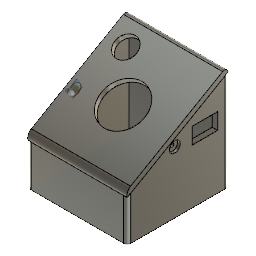
AntiThief_yanweibo (Autodesk Fusion 360 design; units mm, degrees)
Autodesk Fusion 360 part; units mm, degrees
sketch "Sketch1" plane through (0, 0, 0) normal (0, 1, 0) x (1, 0, 0) in component "Case"
  line L0 (27.5, 11.5) -> (-27.5, 11.5)
  line L1 (-27.5, 11.5) -> (-27.5, -11.5)
  line L2 (-27.5, -11.5) -> (27.5, -11.5)
  line L3 (27.5, -11.5) -> (27.5, 11.5)
  line L4 (27.5, 11.5) -> (-27.5, -11.5) construction
  line L5 (-27.5, 11.5) -> (27.5, -11.5) construction
  dimension "d1" = 55
  dimension "d2" = 23
  constraint perpendicular L0 L1
  constraint parallel L0 L2
  constraint parallel L1 L3
  constraint horizontal L0
  constraint coincident L4 origin
  constraint coincident L5 origin
  measures "d1" distance of L1.end L2.end
  measures "d2" distance of L0.end L1.end
extrude "Extrude1" add sketch "Sketch1" along normal blind 56 contours L0 L1 L2 L3 picked at (-9.166667, -3.833333) makes body 1 in component "Case"
sketch "Sketch3" plane through (0, 0, 11.5) normal (0, 0, 1) x (-1, 0, 0) in component "Case"
  line L0 (27.5, 0) -> (-27.5, 0)
  line L1 (-27.5, 0) -> (-27.5, -56)
  line L2 (-27.5, -56) -> (27.5, -56)
  line L3 (27.5, -56) -> (27.5, 0)
  line L4 (24.5, -53) -> (24.5, -3)
  line L5 (24.5, -3) -> (-24.5, -3)
  line L6 (-24.5, -3) -> (-24.5, -53)
  line L7 (-24.5, -53) -> (24.5, -53)
  dimension "d7" = -3
extrude "Extrude2" cut sketch "Sketch3" against normal blind 20 contours L4 L5 L6 L7 picked at (-8.166667, -36.333333) bodies 1 in component "Case"
draft "Draft1" angle 30 neutral plane through (0, 0, 0) pull (0, -1, 0) 1 faces at (-26.5, 36.333333, 11.5) on bodies 1 in component "Case"
sketch "Sketch1 (2)" plane through (0, -4.979646, 8.625) normal (0, -0.5, 0.866025) x (1, 0, 0) in component "Top"
  line L0 (-24.5, 9.214102) -> (-24.5, 66.949129)
  line L1 (-24.5, 66.949129) -> (24.5, 66.949129)
  line L2 (24.5, 66.949129) -> (24.5, 9.214102)
  line L3 (24.5, 9.214102) -> (-24.5, 9.214102)
  line L4 (-27.5, 5.75) -> (27.5, 5.75)
  line L5 (27.5, 5.75) -> (27.5, 70.41323)
  line L6 (27.5, 70.41323) -> (-27.5, 70.41323)
  line L7 (-27.5, 70.41323) -> (-27.5, 5.75)
extrude "Extrude1'" add sketch "Sketch1 (2)" along normal blind 3 separate body contours L4 L5 L6 L7 picked at (-8.166667, 6.904701) makes body 2 in component "Top"
fillet "Fillet1" radius 2 4 edges at (27.5, 56, 16.165808) (27.5, 0, 0) (-27.5, 0, 0) (-27.5, 56, 16.165808) on bodies 1 in component "Case"
fillet "Fillet1'" radius 4 1 edges at (0, -1.5, 14.098076) on bodies 2 in component "Top"
fillet "Fillet2" radius 2 1 edges at (0, 54.5, 46.429691) on bodies 2 in component "Top"
sketch "Sketch5" plane through (0, 0, -8.5) normal (0, 0, 1) x (-1, 0, 0) in component "Case"
  line L0 (-24.5, -53) -> (24.5, -53)
  line L1 (24.5, -53) -> (24.5, -3)
  line L2 (24.5, -3) -> (-24.5, -3)
  line L3 (-24.5, -3) -> (-24.5, -53)
  line L4 (-25, -30) -> (25, -30)
  line L5 (25, -30) -> (25, -33)
  line L6 (25, -33) -> (-25, -33)
  line L7 (-25, -33) -> (-25, -30)
  line L8 (-25, -30) -> (25, -33) construction
  line L9 (25, -30) -> (-25, -33) construction
  line L10 (-25.5, 0) -> (25.5, 0)
  line L11 (-25.5, -56) -> (25.5, -56)
  point P0 (0, -31.5)
  dimension "d15" = 3
  dimension "d16" = 50
  dimension "d17" = 30
  dimension "d18" = 23
  constraint perpendicular L4 L5
  constraint parallel L4 L6
  constraint parallel L5 L7
  constraint horizontal L4
  constraint coincident L8 P0
  constraint coincident L9 P0
  measures "d15" distance of L4.end L5.end
  measures "d16" distance of L5.end L6.end
  measures "d17" distance of L4 L10
  measures "d18" distance of L6.end L11
extrude "Extrude3" add sketch "Sketch5" along normal blind 10 contours L1 L3 L4 L6 picked at (-8.166667, -31) bodies 1 in component "Case"
sketch "Sketch6" plane through (27.5, 0, 0) normal (1, 0, 0) x (0, 1, 0) in component "Case"
  line L0 (2, 12.654701) -> (2, -11.5)
  line L1 (2, -11.5) -> (54, -11.5)
  line L2 (54, -11.5) -> (54, 42.676915)
  line L3 (54, 42.676915) -> (2, 12.654701)
  circle A0 centre (26.320508, 22.654701) radius 3
  line L4 (36, 27.665808) -> (50, 27.665808)
  line L5 (50, 27.665808) -> (50, 18.665808)
  line L6 (50, 18.665808) -> (36, 18.665808)
  line L7 (36, 18.665808) -> (36, 27.665808)
  dimension "d21" = 6
  dimension "d22" = 3.5
  dimension "d23" = 10
  dimension "d92" = 14
  dimension "d93" = 9
  dimension "d94" = 18
  dimension "d95" = 4
  constraint horizontal L4
  constraint vertical L5
  constraint horizontal L6
  constraint vertical L7
  measures "d21" diameter of A0
extrude "Extrude6" cut sketch "Sketch6" against normal blind 3 contours L4 L5 L6 L7 picked at (40.666667, 21.665808) bodies 1 in component "Case"
hole "Hole2" at (27.5, 26.320508, 22.654701) direction (-1, 0, 0) diameter 2 depth 6 tip angle 118 bodies 1 in component "Case"
extrude "Extrude4" cut sketch "Sketch6" against normal blind 1.5 contours A0 picked at (26.245778, 23.519244) bodies 1 in component "Case"
sketch "Sketch8" plane through (-27.5, 0, 0) normal (-1, 0, 0) x (0, -1, 0) in component "Case"
  line L0 (-54, 42.676915) -> (-54, -11.5)
  line L1 (-54, -11.5) -> (-2, -11.5)
  line L2 (-2, -11.5) -> (-2, 12.654701)
  line L3 (-2, 12.654701) -> (-54, 42.676915)
  circle A0 centre (-26.320508, 22.654701) radius 3
  line L4 (-21.944825, 24.169851) -> (-24.944825, 18.973698)
  line L5 (-24.944825, 18.973698) -> (-30.140978, 21.973698)
  line L6 (-30.140978, 21.973698) -> (-27.140978, 27.169851)
  line L7 (-30.140978, 21.973698) -> (-24.125026, 21.973698) construction
  line L8 (-27.140978, 27.169851) -> (-21.944825, 24.169851)
  dimension "d29" = 6
  dimension "d30" = 10
  dimension "d31" = 3.5
  dimension "d53" = 6
  dimension "d54" = 6
  dimension "d55" = 60
  dimension "d56" = 6
  constraint perpendicular L3 L4
  constraint perpendicular L4 L5
  constraint horizontal L7
  measures "d29" diameter of A0
  measures "d55" angle of L6 L7
hole "Hole1" at (-27.5, 26.320508, 22.654701) direction (1, 0, 0) diameter 2 depth 6 tip angle 118 bodies 1 in component "Case"
extrude "Extrude5" cut sketch "Sketch8" against normal blind 1.5 contours A0 L6 | A0 L5 L6 | A0 L5 picked at (-28.923464, 24.10138) picked at (-27.239065, 23.000716) picked at (-27.238076, 20.214879) bodies 1 in component "Case"
sketch "Sketch2" plane through (-24.5, 0, 0) normal (1, 0, 0) x (0, 1, 0) in component "Top"
  arc A0 (1.854102, 16.034568) -> (1.510476, 15.811981) centre (3.854102, 12.570466) ccw
  line L0 (1.510476, 15.811981) -> (3, 13.232051)
  line L1 (3, 13.232051) -> (53, 42.099564)
  line L2 (53, 42.099564) -> (51.5, 44.69764)
  line L3 (51.5, 44.69764) -> (1.854102, 16.034568)
extrude "Extrude2'" add sketch "Sketch2" along normal blind 44 contours A0 L0 L1 L2 L3 picked at (19.284701, 23.788728) bodies 2 in component "Top"
extrude "拉伸8" add 1 faces at (19.5, 19.284701, 23.788728) along direction (1, 0, 0) blind 5 on bodies 2 bodies 2 in component "Top"
sketch "Sketch7" plane through (0, -4.979646, 8.625) normal (0, 0.5, -0.866025) x (-1, 0, 0) in component "Top"
  line L0 (27.5, 5.75) -> (27.5, 70.41323)
  line L1 (27.5, 70.41323) -> (-27.5, 70.41323)
  line L2 (-27.5, 70.41323) -> (-27.5, 5.75)
  line L3 (-27.5, 5.75) -> (27.5, 5.75)
  line L4 (-24.5, 37.13) -> (-19.5, 37.13)
  line L5 (-19.5, 37.13) -> (-19.5, 31.13)
  line L6 (-19.5, 31.13) -> (-24.5, 31.13)
  line L7 (-24.5, 31.13) -> (-24.5, 37.13)
  line L8 (24.5, 37.13) -> (19.5, 37.13)
  line L9 (19.5, 37.13) -> (19.5, 31.13)
  line L10 (19.5, 31.13) -> (24.5, 31.13)
  line L11 (24.5, 31.13) -> (24.5, 37.13)
  dimension "d72" = 5
  dimension "d73" = 6
  dimension "d74" = 3
  dimension "d76" = 6
  dimension "d78" = 3
  dimension "d79" = 25.38
  dimension "d80" = 25.38
  dimension "d100" = 5
  constraint horizontal L4
  constraint vertical L5
  constraint horizontal L6
  constraint vertical L7
  constraint horizontal L8
  constraint vertical L9
  constraint horizontal L10
  constraint vertical L11
  measures "d72" distance of L4.start L4.end
  measures "d73" distance of L4.start L6.end
  measures "d74" distance of L2 L4.start
  measures "d76" distance of L8.start L10.end
  measures "d78" distance of L0 L11
  measures "d79" vertical distance of L2.end L6.end
  measures "d80" distance of L3 L10.end
  measures "d100" distance of L8.start L8.end
extrude "Extrude7" add sketch "Sketch7" along normal blind 7 contours L4 L5 L6 L7 | L8 L9 L10 L11 picked at (-22.833333, 35.13) picked at (21.166667, 35.13) bodies 2 in component "Top"
hole "Hole3" at (24.5, 26.327801, 22.658911) direction (-1, 0, 0) diameter 2 depth 6 tip angle 118 bodies 2 in component "Top"
hole "Hole4" at (-24.5, 26.327801, 22.658911) direction (1, 0, 0) diameter 2 depth 6 tip angle 118 bodies 2 in component "Top"
sketch "Sketch5 (2)" plane through (0, -6.479646, 11.223076) normal (0, -0.5, 0.866025) x (1, 0, 0) in component "Top"
  line L0 (-27.5, 9.622983) -> (27.5, 9.622983)
  line L1 (27.5, 9.622983) -> (27.5, 68.41323)
  line L2 (27.5, 68.41323) -> (-27.5, 68.41323)
  line L3 (-27.5, 68.41323) -> (-27.5, 9.622983)
  circle A0 centre (0, 36.622983) radius 12
  circle A1 centre (-16.5, 57.41323) radius 6
  line L4 (27.5, 70.41323) -> (-27.5, 70.41323)
  dimension "d62" = 24
  dimension "d63" = 27.5
  dimension "d64" = 27
  dimension "d89" = 12
  dimension "d90" = 11
  dimension "d91" = 13
  measures "d62" diameter of A0
  measures "d89" diameter of A1
extrude "Extrude5'" cut sketch "Sketch5 (2)" against normal blind 3 contours A0 | A1 picked at (2.393572, 39.084281) picked at (-15.25302, 58.976893) bodies 2 in component "Top"
component "Top" placed x (1, 0, 0) y (0, 1, 0) z (0, 0, 1) at (0, 0, 0)
component "Case" placed x (1, 0, 0) y (0, 1, 0) z (0, 0, 1) at (0, 0, 0)
